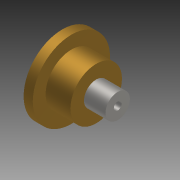
# Autodesk Inventor part: Hitec HS-225MG gear 3
Saved by Autodesk Inventor 2017 SP1 (Build 210196100, 196)
## iProperties
Created: 2018-01-04
Part Number: Hitec HS-225MG gear 3
Material: Generic
Document SubType Name: Modeling
Designer: JT
Density: 1 g/cm^3
Appearance: Default
Author: JT
Autodesk Inventor part; units mm, degrees
ref_plane "YZ Plane" through (0, 0, 0) normal (1, 0, 0) x (0, 1, 0)
ref_plane "XZ Plane" through (0, 0, 0) normal (0, 1, 0) x (-1, 0, 0)
ref_plane "XY Plane" through (0, 0, 0) normal (0, 0, 1) x (1, 0, 0)
sketch "Sketch1" plane through (0, 0, 0) normal (0, 0, 1) x (1, 0, 0)
  line L0 (0, 4.75) -> (0, 5.925)
  line L1 (0, 5.925) -> (1.4, 5.925)
  line L2 (1.4, 5.925) -> (1.4, 3.95)
  line L3 (1.4, 3.95) -> (5.2, 3.95)
  line L4 (5.2, 3.95) -> (5.2, 1.875)
  line L5 (5.2, 1.875) -> (8.5, 1.875)
  line L6 (8.5, 1.875) -> (8.5, 0)
  line L7 (8.5, 0) -> (0, 0)
  line L8 (0, 4.75) -> (0.7, 4.75)
  line L9 (0.7, 4.75) -> (0.7, 2.85)
  line L10 (0.7, 2.85) -> (4, 2.85)
  line L11 (4, 2.85) -> (4, 0)
  dimension "d0" = 8.5
  dimension "d1" = 11.85
  dimension "d2" = 1.4
  dimension "d3" = 5.2
  dimension "d4" = 7.9
  dimension "d5" = 3.75
  dimension "d6" = 9.5
  dimension "d7" = 5.7
  dimension "d8" = 0.7
  dimension "d9" = 4
  constraints: 24 end point, 9 perpendicular, 2 horizontal, 1 point on line, 1 vertical, 1 vertical alignment
  measures "d0" distance from line of L6 L7.end
  measures "d1" diameter of L1 L7
  measures "d2" distance between parallel lines of L2 L0
  measures "d3" distance between parallel lines of L4 L0
  measures "d4" diameter of L3 L7
  measures "d5" diameter of L5 L7
  measures "d6" diameter of L8 L7
  measures "d7" diameter of L10 L7
  measures "d8" distance between parallel lines of L9 L0
  measures "d9" distance from line of L11 L7.end
revolve "Revolution1" add sketch "Sketch1" angle 360 about axis through (8.5, 0, 0) along (-1, 0, 0)
hole "Hole1" at (8.5, 0, 0) direction (-1, 0, 0) diameter 1.2 end through all
body "Solid1"
